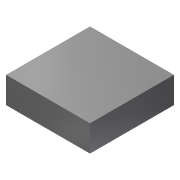
# Autodesk Inventor part: おもり2
Saved by Autodesk Inventor 2013 (Build 170138000, 138)
## iProperties
Created: 2013-12-16
Part Number: おもり2
Material: ステンレス鋼
Document SubType Name: Modeling
Designer: victor
Mass: 661.914 g
Surface Area: 133.12 cm^2
Volume: 81.92 cm^3
Density: 8.08 g/cm^3
Author: victor
Autodesk Inventor part; units mm, degrees
ref_plane "YZ Plane" through (0, 0, 0) normal (1, 0, 0) x (0, 1, 0)
ref_plane "XZ Plane" through (0, 0, 0) normal (0, 1, 0) x (-1, 0, 0)
ref_plane "XY Plane" through (0, 0, 0) normal (0, 0, 1) x (1, 0, 0)
sketch "スケッチ1" plane through (0, 0, 0) normal (0, 0, 1) x (1, 0, 0)
  line L0 (-31.7529, 14.4397) -> (32.2471, 14.4397)
  line L1 (32.2471, 14.4397) -> (32.2471, -49.5603)
  line L2 (32.2471, -49.5603) -> (-31.7529, -49.5603)
  line L3 (-31.7529, -49.5603) -> (-31.7529, 14.4397)
  point P0 (0, 0)
  dimension "d0" = 64
  dimension "d2" = 64
  constraints: 8 end point, 2 parallel, 1 horizontal, 1 perpendicular
  measures "d0" distance of L0.start L0.end
  measures "d2" distance of L2.end L0.start
extrude "押し出し1" add sketch "スケッチ1" along normal blind 20
